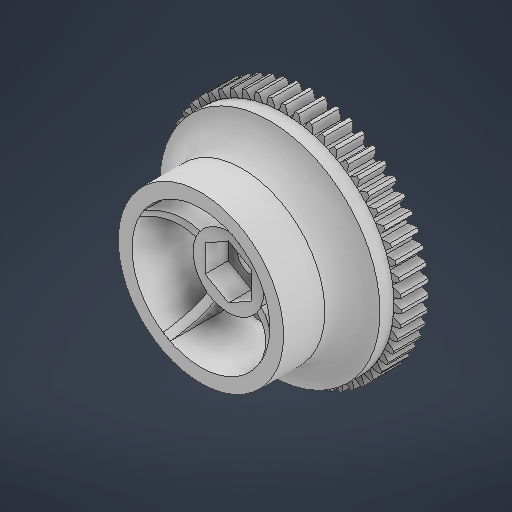
# Autodesk Inventor part: wheel_v4
Saved by Autodesk Inventor 2027.1 (Build 311270010, 270A)
## iProperties
Created: 2026-09-04
Part Number: wheel_v4
Material: Generic
Document SubType Name: Modeling
Designer: ajrcr
Density: 1 g/cm^3
Appearance: Default
Author: ajrcr
Autodesk Inventor part; units mm, degrees
ref_plane "YZ Plane" through (0, 0, 0) normal (1, 0, 0) x (0, 1, 0)
ref_plane "XZ Plane" through (0, 0, 0) normal (0, 1, 0) x (-1, 0, 0)
ref_plane "XY Plane" through (0, 0, 0) normal (0, 0, 1) x (1, 0, 0)
sketch "Sketch1" plane through (0, 0, 0) normal (0, 0, 1) x (1, 0, 0)
  circle A0 centre (0, 0) radius 30
  circle A1 centre (0, 0) radius 40
  circle A2 centre (0, 0) radius 25
  circle A3 centre (0, 0) radius 12.8
  circle A4 centre (0, 0) radius 5.3
  circle A5 centre (0, 0) radius 9.75 construction
  line L0 (0, 9.75) -> (8.4437, 4.875)
  line L1 (8.4437, 4.875) -> (8.4437, -4.875)
  line L2 (8.4437, -4.875) -> (0, -9.75)
  line L3 (0, -9.75) -> (-8.4437, -4.875)
  line L4 (-8.4437, -4.875) -> (-8.4437, 4.875)
  line L5 (-8.4437, 4.875) -> (0, 9.75)
  line L6 (0, 9.75) -> (0, -9.75) construction
  dimension "bolt_head_hub_WAC" = 19.5
  dimension "wheel_diam" = 60
  dimension "d1" = 80
  dimension "d4" = 50
  dimension "d5" = 25.6
  dimension "hub_id" = 10.6
  constraints: 14 end point, 7 coincident, 5 centre point, 1 vertical, 1 vertical alignment, 15 other
  measures "wheel_diam" diameter of A0
  measures "d1" diameter of A1
  measures "d4" diameter of A2
  measures "d5" diameter of A3
  measures "hub_id" diameter of A4
extrude "Extrusion1" add sketch "Sketch1" along normal blind 5 contours A0 | A1 | A2 | A3 | A4 | L0 L1 L2 L3 L4 L5
extrude "Extrusion2" add sketch "Sketch1" along normal blind 30 contours A0
extrude "Extrusion3" add sketch "Sketch1" along normal blind 20 contours A3 | L0 L1 L2 L3 L4 L5
extrude "Extrusion4" cut sketch "Sketch1" against normal blind 8.4 from surface at 20 contours L0 L1 L2 L3 L4 L5
extrude "Extrusion5" cut sketch "Sketch1" along normal up to surface (5 mm away) contours A4
fillet "Fillet1" radius 10 1 edges at (-30, 0, 5)
ref_plane "Work Plane1" through (-8.4437, 4.875, 0) normal (-0.5, -0.8660254, 0) x (0, 0, -1)
sketch "Sketch3" plane through (-8.4437, 4.875, 0) normal (-0.5, -0.8660254, 0) x (0, 0, -1)
  line L0 (-5, 22.55) -> (-20, 22.55) projected
  line L1 (-5, 34.75) -> (-5, -15.25) projected
  line L2 (-5, -3.05) -> (-5, 22.55) projected
  line L3 (-30, 34.75) -> (-5, 34.75) projected
  line L4 (-20, 22.55) -> (-5, 22.55)
  line L5 (-5, 22.55) -> (-5, 19.55)
  line L6 (-5, 19.55) -> (-20, 19.55)
  line L7 (-20, 19.55) -> (-20, 22.55)
  arc A0 (-20, 22.55) -> (-30, 34.75) centre (-34.8676, 20.5618) ccw
  point P0 (0, 9.75)
  dimension "d18" = 3
  dimension "d21" = 15
  constraints: 8 end point, 2 parallel, 2 point on circle, 1 centre point, 1 horizontal, 1 perpendicular, 1 point on line
  measures "d18" distance between parallel lines of L6 L0
  measures "d21" radius of A0
extrude "Extrusion6" add sketch "Sketch3" along normal mid plane 3
pattern_circular "Circular Pattern1" count 4 over 360 about axis through (0, 0, -10) along (0, 0, 1) of "Extrusion6"
sketch "Sketch4" plane through (0, 0, 0) normal (0, 0, -1) x (-1, 0, 0)
  circle A0 centre (0, 0) radius 5.3 projected
  circle A1 centre (0, 0) radius 45
  dimension "d25" = 90
  constraints: 1 centre point, 1 coincident
  measures "d25" diameter of A1
extrude "Extrusion7" add sketch "Sketch4" along normal blind 10
spur gear teeth "Spur Gear1" teeth 55 pitch diameter 82.5 tip diameter 85.5 root diameter 78.75 face width 10 trims to tip circle yes start plane through (0, 0, -10) normal (0, 0, -1) x (-1, 0, 0)
equation "\"bolt_head_hub_WAC\" = bolt_WAC + 2 * printer_tolerance"
equation "\"d1\" = wheel_diam + 2 * flange_extra"
equation "\"d4\" = wheel_diam - 2 * wheel_thick"
equation "\"d5\" = bolt_head_hub_WAC + 2 * bolt_head_hub_clearance"
equation "\"hub_id\" = bolt_od + 2 * printer_tolerance"
equation "\"d8\" = track_w + flange_w"
equation "\"d10\" = flange_w + hub_height"
equation "\"track_w\" = 25"
equation "\"wheel_thick\" = 5"
equation "\"bolt_head_hub_clearance\" = 3.05"
equation "\"hub_height\" = 15"
equation "\"bolt_head_thick\" = 6.4"
equation "\"bolt_WAC\" = 18.9"
equation "\"printer_tolerance\" = 0.3"
equation "\"flange_extra\" = 10"
equation "\"bolt_od\" = 10"
equation "\"flange_w\" = 5"
body "Solid1"
